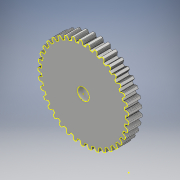
# Autodesk Inventor part: Engranaje_V_G_2
Saved by Autodesk Inventor 2017 (Build 210142000, 142)
## iProperties
Created: 2016-10-02
Part Number: Engranaje_V_G_2
Material: Generic
Document SubType Name: Modeling
Designer: CASA
Density: 1 g/cm^3
Appearance: Default
Author: CASA
Autodesk Inventor part; units mm, degrees
note: some values were not read from the file. Chosen so that the rebuilt part matches the saved one: sketch regions of "Extrusion1".
(part 1 of 2)
ref_plane "YZ Plane" through (0, 0, 0) normal (1, 0, 0) x (0, 1, 0)
ref_plane "XZ Plane" through (0, 0, 0) normal (0, 1, 0) x (-1, 0, 0)
ref_plane "XY Plane" through (0, 0, 0) normal (0, 0, 1) x (1, 0, 0)
sketch "Sketch1" plane through (0, 0, 0) normal (0, 1, 0) x (-1, 0, 0)
  line L0 (1.1447, 1.0054) -> (1.14, 0.9694)
  line L1 (1.14, 0.9694) -> (1.1261, 0.9358)
  line L2 (1.1261, 0.9358) -> (1.104, 0.907)
  line L3 (1.104, 0.907) -> (1.0751, 0.8848)
  line L4 (1.0751, 0.8848) -> (1.0415, 0.8709)
  line L5 (1.0415, 0.8709) -> (1.0055, 0.8662)
  line L6 (1.0055, 0.8662) -> (0.9694, 0.8709)
  line L7 (0.9694, 0.8709) -> (0.9358, 0.8848)
  line L8 (0.9358, 0.8848) -> (0.907, 0.907)
  line L9 (0.907, 0.907) -> (0.8848, 0.9358)
  line L10 (0.8848, 0.9358) -> (0.8709, 0.9694)
  line L11 (0.8709, 0.9694) -> (0.8662, 1.0055)
  line L12 (0.8662, 1.0055) -> (0.8709, 1.0415)
  line L13 (0.8709, 1.0415) -> (0.8848, 1.0751)
  line L14 (0.8848, 1.0751) -> (0.907, 1.104)
  line L15 (0.907, 1.104) -> (0.9358, 1.1261)
  line L16 (0.9358, 1.1261) -> (0.9694, 1.14)
  line L17 (0.9694, 1.14) -> (1.0055, 1.1447)
  line L18 (1.0055, 1.1447) -> (1.0415, 1.14)
  line L19 (1.0415, 1.14) -> (1.0751, 1.1261)
  line L20 (1.0751, 1.1261) -> (1.104, 1.104)
  line L21 (1.104, 1.104) -> (1.1261, 1.0751)
  line L22 (1.1261, 1.0751) -> (1.14, 1.0415)
  line L23 (1.14, 1.0415) -> (1.1447, 1.0054)
  line L24 (1.935, 1.0367) -> (1.9383, 1.036)
  line L25 (1.9383, 1.036) -> (1.9449, 1.0346)
  line L26 (1.9449, 1.0346) -> (1.9582, 1.0311)
  line L27 (1.9582, 1.0311) -> (1.9714, 1.0269)
  line L28 (1.9714, 1.0269) -> (1.9846, 1.0221)
  line L29 (1.9846, 1.0221) -> (1.9978, 1.0168)
  line L30 (1.9978, 1.0168) -> (2.0109, 1.0108)
  line L31 (2.0109, 1.0108) -> (2.0098, 0.9593)
  line L32 (2.0098, 0.9593) -> (1.9964, 0.9539)
  line L33 (1.9964, 0.9539) -> (1.983, 0.9491)
  line L34 (1.983, 0.9491) -> (1.9696, 0.9449)
  line L35 (1.9696, 0.9449) -> (1.9562, 0.9412)
  line L36 (1.9562, 0.9412) -> (1.9429, 0.9383)
  line L37 (1.9429, 0.9383) -> (1.9362, 0.9371)
  line L38 (1.9362, 0.9371) -> (1.9329, 0.9366)
  line L39 (1.9329, 0.9366) -> (1.9296, 0.9361)
  line L40 (1.9296, 0.9361) -> (1.9237, 0.8803)
  line L41 (1.9237, 0.8803) -> (1.9268, 0.8792)
  line L42 (1.9268, 0.8792) -> (1.93, 0.878)
  line L43 (1.93, 0.878) -> (1.9363, 0.8754)
  line L44 (1.9363, 0.8754) -> (1.9487, 0.8698)
  line L45 (1.9487, 0.8698) -> (1.961, 0.8634)
  line L46 (1.961, 0.8634) -> (1.9732, 0.8565)
  line L47 (1.9732, 0.8565) -> (1.9853, 0.849)
  line L48 (1.9853, 0.849) -> (1.9973, 0.8409)
  line L49 (1.9973, 0.8409) -> (1.9876, 0.7902)
  line L50 (1.9876, 0.7902) -> (1.9735, 0.7872)
  line L51 (1.9735, 0.7872) -> (1.9595, 0.7847)
  line L52 (1.9595, 0.7847) -> (1.9455, 0.7828)
  line L53 (1.9455, 0.7828) -> (1.9317, 0.7815)
  line L54 (1.9317, 0.7815) -> (1.9181, 0.7808)
  line L55 (1.9181, 0.7808) -> (1.9113, 0.7808)
  line L56 (1.9113, 0.7808) -> (1.9079, 0.7808)
  line L57 (1.9079, 0.7808) -> (1.9046, 0.7809)
  line L58 (1.9046, 0.7809) -> (1.8893, 0.727)
  line L59 (1.8893, 0.727) -> (1.8923, 0.7253)
  line L60 (1.8923, 0.7253) -> (1.8952, 0.7236)
  line L61 (1.8952, 0.7236) -> (1.9009, 0.72)
  line L62 (1.9009, 0.72) -> (1.9122, 0.7123)
  line L63 (1.9122, 0.7123) -> (1.9233, 0.704)
  line L64 (1.9233, 0.704) -> (1.9342, 0.6951)
  line L65 (1.9342, 0.6951) -> (1.9448, 0.6856)
  line L66 (1.9448, 0.6856) -> (1.9553, 0.6757)
  line L67 (1.9553, 0.6757) -> (1.9371, 0.6273)
  line L68 (1.9371, 0.6273) -> (1.9226, 0.6267)
  line L69 (1.9226, 0.6267) -> (1.9084, 0.6267)
  line L70 (1.9084, 0.6267) -> (1.8944, 0.6271)
  line L71 (1.8944, 0.6271) -> (1.8805, 0.6282)
  line L72 (1.8805, 0.6282) -> (1.8669, 0.6298)
  line L73 (1.8669, 0.6298) -> (1.8603, 0.6309)
  line L74 (1.8603, 0.6309) -> (1.857, 0.6316)
  line L75 (1.857, 0.6316) -> (1.8537, 0.6322)
  line L76 (1.8537, 0.6322) -> (1.8295, 0.5816)
  line L77 (1.8295, 0.5816) -> (1.8321, 0.5795)
  line L78 (1.8321, 0.5795) -> (1.8347, 0.5773)
  line L79 (1.8347, 0.5773) -> (1.8397, 0.5728)
  line L80 (1.8397, 0.5728) -> (1.8496, 0.5633)
  line L81 (1.8496, 0.5633) -> (1.8591, 0.5532)
  line L82 (1.8591, 0.5532) -> (1.8683, 0.5426)
  line L83 (1.8683, 0.5426) -> (1.8772, 0.5315)
  line L84 (1.8772, 0.5315) -> (1.8858, 0.5199)
  line L85 (1.8858, 0.5199) -> (1.8597, 0.4753)
  line L86 (1.8597, 0.4753) -> (1.8454, 0.4772)
  line L87 (1.8454, 0.4772) -> (1.8314, 0.4795)
  line L88 (1.8314, 0.4795) -> (1.8176, 0.4823)
  line L89 (1.8176, 0.4823) -> (1.8042, 0.4857)
  line L90 (1.8042, 0.4857) -> (1.7911, 0.4896)
  line L91 (1.7911, 0.4896) -> (1.7847, 0.4919)
  line L92 (1.7847, 0.4919) -> (1.7815, 0.493)
  line L93 (1.7815, 0.493) -> (1.7784, 0.4942)
  line L94 (1.7784, 0.4942) -> (1.746, 0.4484)
  line L95 (1.746, 0.4484) -> (1.7482, 0.4459)
  line L96 (1.7482, 0.4459) -> (1.7504, 0.4433)
  line L97 (1.7504, 0.4433) -> (1.7546, 0.438)
  line L98 (1.7546, 0.438) -> (1.7627, 0.427)
  line L99 (1.7627, 0.427) -> (1.7704, 0.4154)
  line L100 (1.7704, 0.4154) -> (1.7776, 0.4034)
  line L101 (1.7776, 0.4034) -> (1.7845, 0.391)
  line L102 (1.7845, 0.391) -> (1.7911, 0.3781)
  line L103 (1.7911, 0.3781) -> (1.7578, 0.3386)
  line L104 (1.7578, 0.3386) -> (1.744, 0.3428)
  line L105 (1.744, 0.3428) -> (1.7306, 0.3475)
  line L106 (1.7306, 0.3475) -> (1.7175, 0.3526)
  line L107 (1.7175, 0.3526) -> (1.7048, 0.3582)
  line L108 (1.7048, 0.3582) -> (1.6926, 0.3643)
  line L109 (1.6926, 0.3643) -> (1.6866, 0.3676)
  line L110 (1.6866, 0.3676) -> (1.6837, 0.3692)
  line L111 (1.6837, 0.3692) -> (1.6808, 0.371)
  line L112 (1.6808, 0.371) -> (1.6412, 0.3313)
  line L113 (1.6412, 0.3313) -> (1.6429, 0.3284)
  line L114 (1.6429, 0.3284) -> (1.6446, 0.3255)
  line L115 (1.6446, 0.3255) -> (1.6479, 0.3196)
  line L116 (1.6479, 0.3196) -> (1.654, 0.3073)
  line L117 (1.654, 0.3073) -> (1.6596, 0.2947)
  line L118 (1.6596, 0.2947) -> (1.6648, 0.2816)
  line L119 (1.6648, 0.2816) -> (1.6695, 0.2681)
  line L120 (1.6695, 0.2681) -> (1.6737, 0.2543)
  line L121 (1.6737, 0.2543) -> (1.6343, 0.221)
  line L122 (1.6343, 0.221) -> (1.6214, 0.2275)
  line L123 (1.6214, 0.2275) -> (1.6089, 0.2344)
  line L124 (1.6089, 0.2344) -> (1.5969, 0.2417)
  line L125 (1.5969, 0.2417) -> (1.5853, 0.2493)
  line L126 (1.5853, 0.2493) -> (1.5743, 0.2574)
  line L127 (1.5743, 0.2574) -> (1.569, 0.2616)
  line L128 (1.569, 0.2616) -> (1.5664, 0.2638)
  line L129 (1.5664, 0.2638) -> (1.5639, 0.266)
  line L130 (1.5639, 0.266) -> (1.5181, 0.2335)
  line L131 (1.5181, 0.2335) -> (1.5193, 0.2304)
  line L132 (1.5193, 0.2304) -> (1.5205, 0.2273)
  line L133 (1.5205, 0.2273) -> (1.5227, 0.2209)
  line L134 (1.5227, 0.2209) -> (1.5267, 0.2078)
  line L135 (1.5267, 0.2078) -> (1.5301, 0.1943)
  line L136 (1.5301, 0.1943) -> (1.5329, 0.1806)
  line L137 (1.5329, 0.1806) -> (1.5353, 0.1665)
  line L138 (1.5353, 0.1665) -> (1.5372, 0.1522)
  line L139 (1.5372, 0.1522) -> (1.4927, 0.126)
  line L140 (1.4927, 0.126) -> (1.4811, 0.1346)
  line L141 (1.4811, 0.1346) -> (1.4699, 0.1435)
  line L142 (1.4699, 0.1435) -> (1.4593, 0.1527)
  line L143 (1.4593, 0.1527) -> (1.4492, 0.1622)
  line L144 (1.4492, 0.1622) -> (1.4397, 0.172)
  line L145 (1.4397, 0.172) -> (1.4352, 0.1771)
  line L146 (1.4352, 0.1771) -> (1.433, 0.1796)
  line L147 (1.433, 0.1796) -> (1.4309, 0.1822)
  line L148 (1.4309, 0.1822) -> (1.3803, 0.158)
  line L149 (1.3803, 0.158) -> (1.3809, 0.1547)
  line L150 (1.3809, 0.1547) -> (1.3816, 0.1514)
  line L151 (1.3816, 0.1514) -> (1.3827, 0.1447)
  line L152 (1.3827, 0.1447) -> (1.3844, 0.1312)
  line L153 (1.3844, 0.1312) -> (1.3854, 0.1173)
  line L154 (1.3854, 0.1173) -> (1.3859, 0.1033)
  line L155 (1.3859, 0.1033) -> (1.3859, 0.089)
  line L156 (1.3859, 0.089) -> (1.3853, 0.0746)
  line L157 (1.3853, 0.0746) -> (1.337, 0.0563)
  line L158 (1.337, 0.0563) -> (1.327, 0.0668)
  line L159 (1.327, 0.0668) -> (1.3176, 0.0774)
  line L160 (1.3176, 0.0774) -> (1.3086, 0.0883)
  line L161 (1.3086, 0.0883) -> (1.3003, 0.0993)
  line L162 (1.3003, 0.0993) -> (1.2926, 0.1106)
  line L163 (1.2926, 0.1106) -> (1.289, 0.1164)
  line L164 (1.289, 0.1164) -> (1.2873, 0.1193)
  line L165 (1.2873, 0.1193) -> (1.2856, 0.1222)
  line L166 (1.2856, 0.1222) -> (1.2316, 0.1068)
  line L167 (1.2316, 0.1068) -> (1.2318, 0.1035)
  line L168 (1.2318, 0.1035) -> (1.2318, 0.1001)
  line L169 (1.2318, 0.1001) -> (1.2318, 0.0934)
  line L170 (1.2318, 0.0934) -> (1.2312, 0.0797)
  line L171 (1.2312, 0.0797) -> (1.2299, 0.0659)
  line L172 (1.2299, 0.0659) -> (1.228, 0.052)
  line L173 (1.228, 0.052) -> (1.2255, 0.0379)
  line L174 (1.2255, 0.0379) -> (1.2225, 0.0238)
  line L175 (1.2225, 0.0238) -> (1.1718, 0.014)
  line L176 (1.1718, 0.014) -> (1.1638, 0.0259)
  line L177 (1.1638, 0.0259) -> (1.1562, 0.038)
  line L178 (1.1562, 0.038) -> (1.1492, 0.0502)
  line L179 (1.1492, 0.0502) -> (1.1429, 0.0625)
  line L180 (1.1429, 0.0625) -> (1.1372, 0.075)
  line L181 (1.1372, 0.075) -> (1.1346, 0.0812)
  line L182 (1.1346, 0.0812) -> (1.1334, 0.0844)
  line L183 (1.1334, 0.0844) -> (1.1323, 0.0875)
  line L184 (1.1323, 0.0875) -> (1.0765, 0.0815)
  line L185 (1.0765, 0.0815) -> (1.076, 0.0782)
  line L186 (1.076, 0.0782) -> (1.0755, 0.0749)
  line L187 (1.0755, 0.0749) -> (1.0744, 0.0682)
  line L188 (1.0744, 0.0682) -> (1.0714, 0.0548)
  line L189 (1.0714, 0.0548) -> (1.0678, 0.0415)
  line L190 (1.0678, 0.0415) -> (1.0636, 0.028)
  line L191 (1.0636, 0.028) -> (1.0588, 0.0146)
  line L192 (1.0588, 0.0146) -> (1.0535, 0.0012)
  line L193 (1.0535, 0.0012) -> (1.0019, 0.0001)
  line L194 (1.0019, 0.0001) -> (0.9959, 0.0132)
  line L195 (0.9959, 0.0132) -> (0.9905, 0.0264)
  line L196 (0.9905, 0.0264) -> (0.9857, 0.0396)
  line L197 (0.9857, 0.0396) -> (0.9815, 0.0528)
  line L198 (0.9815, 0.0528) -> (0.978, 0.0661)
  line L199 (0.978, 0.0661) -> (0.9765, 0.0727)
  line L200 (0.9765, 0.0727) -> (0.9759, 0.076)
  line L201 (0.9759, 0.076) -> (0.9753, 0.0793)
  line L202 (0.9753, 0.0793) -> (0.9193, 0.0828)
  line L203 (0.9193, 0.0828) -> (0.9183, 0.0796)
  line L204 (0.9183, 0.0796) -> (0.9172, 0.0764)
  line L205 (0.9172, 0.0764) -> (0.9149, 0.07)
  line L206 (0.9149, 0.07) -> (0.9098, 0.0573)
  line L207 (0.9098, 0.0573) -> (0.904, 0.0448)
  line L208 (0.904, 0.0448) -> (0.8976, 0.0323)
  line L209 (0.8976, 0.0323) -> (0.8906, 0.0198)
  line L210 (0.8906, 0.0198) -> (0.883, 0.0075)
  line L211 (0.883, 0.0075) -> (0.832, 0.0151)
  line L212 (0.832, 0.0151) -> (0.8284, 0.0291)
  line L213 (0.8284, 0.0291) -> (0.8253, 0.043)
  line L214 (0.8253, 0.043) -> (0.8228, 0.0568)
  line L215 (0.8228, 0.0568) -> (0.8209, 0.0706)
  line L216 (0.8209, 0.0706) -> (0.8197, 0.0842)
  line L217 (0.8197, 0.0842) -> (0.8193, 0.0909)
  line L218 (0.8193, 0.0909) -> (0.8192, 0.0943)
  line L219 (0.8192, 0.0943) -> (0.8192, 0.0977)
  line L220 (0.8192, 0.0977) -> (0.7646, 0.1106)
  line L221 (0.7646, 0.1106) -> (0.7631, 0.1076)
  line L222 (0.7631, 0.1076) -> (0.7615, 0.1046)
  line L223 (0.7615, 0.1046) -> (0.7581, 0.0987)
  line L224 (0.7581, 0.0987) -> (0.751, 0.0871)
  line L225 (0.751, 0.0871) -> (0.7431, 0.0757)
  line L226 (0.7431, 0.0757) -> (0.7347, 0.0645)
  line L227 (0.7347, 0.0645) -> (0.7257, 0.0534)
  line L228 (0.7257, 0.0534) -> (0.7161, 0.0426)
  line L229 (0.7161, 0.0426) -> (0.6671, 0.0587)
  line L230 (0.6671, 0.0587) -> (0.6659, 0.0731)
  line L231 (0.6659, 0.0731) -> (0.6652, 0.0873)
  line L232 (0.6652, 0.0873) -> (0.6651, 0.1013)
  line L233 (0.6651, 0.1013) -> (0.6655, 0.1152)
  line L234 (0.6655, 0.1152) -> (0.6666, 0.1288)
  line L235 (0.6666, 0.1288) -> (0.6674, 0.1355)
  line L236 (0.6674, 0.1355) -> (0.6679, 0.1389)
  line L237 (0.6679, 0.1389) -> (0.6684, 0.1422)
  line L238 (0.6684, 0.1422) -> (0.6168, 0.1641)
  line L239 (0.6168, 0.1641) -> (0.6148, 0.1615)
  line L240 (0.6148, 0.1615) -> (0.6127, 0.1588)
  line L241 (0.6127, 0.1588) -> (0.6085, 0.1536)
  line L242 (0.6085, 0.1536) -> (0.5994, 0.1433)
  line L243 (0.5994, 0.1433) -> (0.5897, 0.1334)
  line L244 (0.5897, 0.1334) -> (0.5795, 0.1238)
  line L245 (0.5795, 0.1238) -> (0.5688, 0.1144)
  line L246 (0.5688, 0.1144) -> (0.5576, 0.1053)
  line L247 (0.5576, 0.1053) -> (0.512, 0.1294)
  line L248 (0.512, 0.1294) -> (0.5132, 0.1438)
  line L249 (0.5132, 0.1438) -> (0.5149, 0.158)
  line L250 (0.5149, 0.158) -> (0.5172, 0.1718)
  line L251 (0.5172, 0.1718) -> (0.5199, 0.1854)
  line L252 (0.5199, 0.1854) -> (0.5233, 0.1987)
  line L253 (0.5233, 0.1987) -> (0.5253, 0.2052)
  line L254 (0.5253, 0.2052) -> (0.5263, 0.2084)
  line L255 (0.5263, 0.2084) -> (0.5274, 0.2115)
  line L256 (0.5274, 0.2115) -> (0.4802, 0.2419)
  line L257 (0.4802, 0.2419) -> (0.4778, 0.2396)
  line L258 (0.4778, 0.2396) -> (0.4753, 0.2373)
  line L259 (0.4753, 0.2373) -> (0.4702, 0.2329)
  line L260 (0.4702, 0.2329) -> (0.4595, 0.2243)
  line L261 (0.4595, 0.2243) -> (0.4483, 0.2162)
  line L262 (0.4483, 0.2162) -> (0.4366, 0.2084)
  line L263 (0.4366, 0.2084) -> (0.4244, 0.201)
  line L264 (0.4244, 0.201) -> (0.4119, 0.1939)
  line L265 (0.4119, 0.1939) -> (0.371, 0.2254)
  line L266 (0.371, 0.2254) -> (0.3746, 0.2394)
  line L267 (0.3746, 0.2394) -> (0.3787, 0.2531)
  line L268 (0.3787, 0.2531) -> (0.3833, 0.2664)
  line L269 (0.3833, 0.2664) -> (0.3883, 0.2793)
  line L270 (0.3883, 0.2793) -> (0.3939, 0.2918)
  line L271 (0.3939, 0.2918) -> (0.3969, 0.2978)
  line L272 (0.3969, 0.2978) -> (0.3985, 0.3008)
  line L273 (0.3985, 0.3008) -> (0.4001, 0.3037)
  line L274 (0.4001, 0.3037) -> (0.3587, 0.3417)
  line L275 (0.3587, 0.3417) -> (0.3559, 0.3398)
  line L276 (0.3559, 0.3398) -> (0.3531, 0.338)
  line L277 (0.3531, 0.338) -> (0.3473, 0.3345)
  line L278 (0.3473, 0.3345) -> (0.3354, 0.3278)
  line L279 (0.3354, 0.3278) -> (0.3229, 0.3217)
  line L280 (0.3229, 0.3217) -> (0.3101, 0.316)
  line L281 (0.3101, 0.316) -> (0.2969, 0.3108)
  line L282 (0.2969, 0.3108) -> (0.2832, 0.3059)
  line L283 (0.2832, 0.3059) -> (0.2483, 0.3439)
  line L284 (0.2483, 0.3439) -> (0.2543, 0.357)
  line L285 (0.2543, 0.357) -> (0.2606, 0.3698)
  line L286 (0.2606, 0.3698) -> (0.2673, 0.3821)
  line L287 (0.2673, 0.3821) -> (0.2745, 0.394)
  line L288 (0.2745, 0.394) -> (0.2821, 0.4054)
  line L289 (0.2821, 0.4054) -> (0.2861, 0.4108)
  line L290 (0.2861, 0.4108) -> (0.2881, 0.4135)
  line L291 (0.2881, 0.4135) -> (0.2902, 0.4161)
  line L292 (0.2902, 0.4161) -> (0.2559, 0.4605)
  line L293 (0.2559, 0.4605) -> (0.2528, 0.4592)
  line L294 (0.2528, 0.4592) -> (0.2497, 0.4578)
  line L295 (0.2497, 0.4578) -> (0.2434, 0.4553)
  line L296 (0.2434, 0.4553) -> (0.2305, 0.4508)
  line L297 (0.2305, 0.4508) -> (0.2172, 0.4469)
  line L298 (0.2172, 0.4469) -> (0.2036, 0.4434)
  line L299 (0.2036, 0.4434) -> (0.1896, 0.4405)
  line L300 (0.1896, 0.4405) -> (0.1754, 0.438)
  line L301 (0.1754, 0.438) -> (0.1474, 0.4814)
  line L302 (0.1474, 0.4814) -> (0.1555, 0.4933)
  line L303 (0.1555, 0.4933) -> (0.1639, 0.5048)
  line L304 (0.1639, 0.5048) -> (0.1726, 0.5158)
  line L305 (0.1726, 0.5158) -> (0.1817, 0.5263)
  line L306 (0.1817, 0.5263) -> (0.1911, 0.5363)
  line L307 (0.1911, 0.5363) -> (0.1959, 0.541)
  line L308 (0.1959, 0.541) -> (0.1984, 0.5433)
  line L309 (0.1984, 0.5433) -> (0.2009, 0.5455)
  line L310 (0.2009, 0.5455) -> (0.1745, 0.595)
  line L311 (0.1745, 0.595) -> (0.1713, 0.5942)
  line L312 (0.1713, 0.5942) -> (0.168, 0.5934)
  line L313 (0.168, 0.5934) -> (0.1614, 0.592)
  line L314 (0.1614, 0.592) -> (0.1479, 0.5898)
  line L315 (0.1479, 0.5898) -> (0.1341, 0.5881)
  line L316 (0.1341, 0.5881) -> (0.1201, 0.587)
  line L317 (0.1201, 0.587) -> (0.1059, 0.5865)
  line L318 (0.1059, 0.5865) -> (0.0915, 0.5865)
  line L319 (0.0915, 0.5865) -> (0.0712, 0.6339)
  line L320 (0.0712, 0.6339) -> (0.0812, 0.6443)
  line L321 (0.0812, 0.6443) -> (0.0914, 0.6543)
  line L322 (0.0914, 0.6543) -> (0.1018, 0.6636)
  line L323 (0.1018, 0.6636) -> (0.1125, 0.6725)
  line L324 (0.1125, 0.6725) -> (0.1235, 0.6806)
  line L325 (0.1235, 0.6806) -> (0.1291, 0.6845)
  line L326 (0.1291, 0.6845) -> (0.1319, 0.6863)
  line L327 (0.1319, 0.6863) -> (0.1347, 0.6881)
  line L328 (0.1347, 0.6881) -> (0.1171, 0.7414)
  line L329 (0.1171, 0.7414) -> (0.1138, 0.7411)
  line L330 (0.1138, 0.7411) -> (0.1104, 0.7409)
  line L331 (0.1104, 0.7409) -> (0.1037, 0.7406)
  line L332 (0.1037, 0.7406) -> (0.09, 0.7407)
  line L333 (0.09, 0.7407) -> (0.0761, 0.7414)
  line L334 (0.0761, 0.7414) -> (0.0621, 0.7427)
  line L335 (0.0621, 0.7427) -> (0.048, 0.7446)
  line L336 (0.048, 0.7446) -> (0.0338, 0.747)
  line L337 (0.0338, 0.747) -> (0.0218, 0.7972)
  line L338 (0.0218, 0.7972) -> (0.0334, 0.8057)
  line L339 (0.0334, 0.8057) -> (0.0452, 0.8138)
  line L340 (0.0452, 0.8138) -> (0.0571, 0.8213)
  line L341 (0.0571, 0.8213) -> (0.0691, 0.8282)
  line L342 (0.0691, 0.8282) -> (0.0813, 0.8344)
  line L343 (0.0813, 0.8344) -> (0.0874, 0.8372)
  line L344 (0.0874, 0.8372) -> (0.0905, 0.8385)
  line L345 (0.0905, 0.8385) -> (0.0936, 0.8398)
  line L346 (0.0936, 0.8398) -> (0.0853, 0.8953)
  line L347 (0.0853, 0.8953) -> (0.0819, 0.8956)
  line L348 (0.0819, 0.8956) -> (0.0786, 0.896)
  line L349 (0.0786, 0.896) -> (0.0719, 0.8969)
  line L350 (0.0719, 0.8969) -> (0.0584, 0.8992)
  line L351 (0.0584, 0.8992) -> (0.0449, 0.9022)
  line L352 (0.0449, 0.9022) -> (0.0313, 0.9059)
  line L353 (0.0313, 0.9059) -> (0.0177, 0.9101)
  line L354 (0.0177, 0.9101) -> (0.0041, 0.9149)
  line L355 (0.0041, 0.9149) -> (0.0008, 0.9664)
  line L356 (0.0008, 0.9664) -> (0.0137, 0.9729)
  line L357 (0.0137, 0.9729) -> (0.0266, 0.9788)
  line L358 (0.0266, 0.9788) -> (0.0396, 0.9842)
  line L359 (0.0396, 0.9842) -> (0.0526, 0.9889)
  line L360 (0.0526, 0.9889) -> (0.0657, 0.993)
  line L361 (0.0657, 0.993) -> (0.0722, 0.9948)
  line L362 (0.0722, 0.9948) -> (0.0755, 0.9955)
  line L363 (0.0755, 0.9955) -> (0.0788, 0.9963)
  line L364 (0.0788, 0.9963) -> (0.0799, 1.0524)
  line L365 (0.0799, 1.0524) -> (0.0767, 1.0533)
  line L366 (0.0767, 1.0533) -> (0.0734, 1.0542)
  line L367 (0.0734, 1.0542) -> (0.067, 1.0562)
  line L368 (0.067, 1.0562) -> (0.0541, 1.0608)
  line L369 (0.0541, 1.0608) -> (0.0413, 1.0661)
  line L370 (0.0413, 1.0661) -> (0.0285, 1.072)
  line L371 (0.0285, 1.072) -> (0.0158, 1.0784)
  line L372 (0.0158, 1.0784) -> (0.0032, 1.0854)
  line L373 (0.0032, 1.0854) -> (0.0086, 1.1368)
  line L374 (0.0086, 1.1368) -> (0.0224, 1.141)
  line L375 (0.0224, 1.141) -> (0.0362, 1.1446)
  line L376 (0.0362, 1.1446) -> (0.0499, 1.1477)
  line L377 (0.0499, 1.1477) -> (0.0635, 1.1502)
  line L378 (0.0635, 1.1502) -> (0.0771, 1.152)
  line L379 (0.0771, 1.152) -> (0.0838, 1.1526)
  line L380 (0.0838, 1.1526) -> (0.0872, 1.1529)
  line L381 (0.0872, 1.1529) -> (0.0905, 1.153)
  line L382 (0.0905, 1.153) -> (0.1011, 1.2081)
  line L383 (0.1011, 1.2081) -> (0.0981, 1.2095)
  line L384 (0.0981, 1.2095) -> (0.0951, 1.211)
  line L385 (0.0951, 1.211) -> (0.089, 1.2141)
  line L386 (0.089, 1.2141) -> (0.0771, 1.2208)
  line L387 (0.0771, 1.2208) -> (0.0654, 1.2281)
  line L388 (0.0654, 1.2281) -> (0.0538, 1.2361)
  line L389 (0.0538, 1.2361) -> (0.0424, 1.2446)
  line L390 (0.0424, 1.2446) -> (0.0311, 1.2537)
  line L391 (0.0311, 1.2537) -> (0.0451, 1.3033)
  line L392 (0.0451, 1.3033) -> (0.0595, 1.3052)
  line L393 (0.0595, 1.3052) -> (0.0736, 1.3065)
  line L394 (0.0736, 1.3065) -> (0.0877, 1.3072)
  line L395 (0.0877, 1.3072) -> (0.1015, 1.3073)
  line L396 (0.1015, 1.3073) -> (0.1152, 1.3068)
  line L397 (0.1152, 1.3068) -> (0.122, 1.3063)
  line L398 (0.122, 1.3063) -> (0.1253, 1.3059)
  line L399 (0.1253, 1.3059) -> (0.1286, 1.3055)
  line L400 (0.1286, 1.3055) -> (0.1484, 1.358)
  line L401 (0.1484, 1.358) -> (0.1456, 1.3599)
  line L402 (0.1456, 1.3599) -> (0.1429, 1.3619)
  line L403 (0.1429, 1.3619) -> (0.1375, 1.3659)
  line L404 (0.1375, 1.3659) -> (0.1269, 1.3746)
  line L405 (0.1269, 1.3746) -> (0.1165, 1.3838)
  line L406 (0.1165, 1.3838) -> (0.1065, 1.3936)
  line L407 (0.1065, 1.3936) -> (0.0966, 1.4039)
  line L408 (0.0966, 1.4039) -> (0.0871, 1.4148)
  line L409 (0.0871, 1.4148) -> (0.1093, 1.4613)
  line L410 (0.1093, 1.4613) -> (0.1237, 1.4607)
  line L411 (0.1237, 1.4607) -> (0.1379, 1.4596)
  line L412 (0.1379, 1.4596) -> (0.1519, 1.458)
  line L413 (0.1519, 1.458) -> (0.1656, 1.4557)
  line L414 (0.1656, 1.4557) -> (0.1789, 1.4529)
  line L415 (0.1789, 1.4529) -> (0.1855, 1.4513)
  line L416 (0.1855, 1.4513) -> (0.1887, 1.4504)
  line L417 (0.1887, 1.4504) -> (0.192, 1.4494)
  line L418 (0.192, 1.4494) -> (0.2203, 1.4978)
  line L419 (0.2203, 1.4978) -> (0.2179, 1.5002)
  line L420 (0.2179, 1.5002) -> (0.2155, 1.5025)
  line L421 (0.2155, 1.5025) -> (0.2109, 1.5075)
  line L422 (0.2109, 1.5075) -> (0.2019, 1.5177)
  line L423 (0.2019, 1.5177) -> (0.1933, 1.5286)
  line L424 (0.1933, 1.5286) -> (0.185, 1.54)
  line L425 (0.185, 1.54) -> (0.1771, 1.5518)
  line L426 (0.1771, 1.5518) -> (0.1695, 1.5641)
  line L427 (0.1695, 1.5641) -> (0.1992, 1.6062)
  line L428 (0.1992, 1.6062) -> (0.2133, 1.6032)
  line L429 (0.2133, 1.6032) -> (0.2271, 1.5997)
  line L430 (0.2271, 1.5997) -> (0.2406, 1.5957)
  line L431 (0.2406, 1.5957) -> (0.2537, 1.5912)
  line L432 (0.2537, 1.5912) -> (0.2665, 1.5862)
  line L433 (0.2665, 1.5862) -> (0.2726, 1.5834)
  line L434 (0.2726, 1.5834) -> (0.2757, 1.582)
  line L435 (0.2757, 1.582) -> (0.2787, 1.5805)
  line L436 (0.2787, 1.5805) -> (0.3148, 1.6234)
  line L437 (0.3148, 1.6234) -> (0.3128, 1.6261)
  line L438 (0.3128, 1.6261) -> (0.3109, 1.6289)
  line L439 (0.3109, 1.6289) -> (0.3071, 1.6345)
  line L440 (0.3071, 1.6345) -> (0.3, 1.6462)
  line L441 (0.3, 1.6462) -> (0.2933, 1.6583)
  line L442 (0.2933, 1.6583) -> (0.2871, 1.6709)
  line L443 (0.2871, 1.6709) -> (0.2813, 1.6839)
  line L444 (0.2813, 1.6839) -> (0.2759, 1.6973)
  line L445 (0.2759, 1.6973) -> (0.3123, 1.7339)
  line L446 (0.3123, 1.7339) -> (0.3257, 1.7285)
  line L447 (0.3257, 1.7285) -> (0.3388, 1.7227)
  line L448 (0.3388, 1.7227) -> (0.3514, 1.7165)
  line L449 (0.3514, 1.7165) -> (0.3635, 1.7098)
  line L450 (0.3635, 1.7098) -> (0.3752, 1.7027)
  line L451 (0.3752, 1.7027) -> (0.3809, 1.699)
  line L452 (0.3809, 1.699) -> (0.3836, 1.697)
  line L453 (0.3836, 1.697) -> (0.3863, 1.6951)
  line L454 (0.3863, 1.6951) -> (0.4292, 1.7313)
  line L455 (0.4292, 1.7313) -> (0.4277, 1.7343)
  line L456 (0.4277, 1.7343) -> (0.4263, 1.7373)
  line L457 (0.4263, 1.7373) -> (0.4235, 1.7435)
  line L458 (0.4235, 1.7435) -> (0.4184, 1.7562)
  line L459 (0.4184, 1.7562) -> (0.4139, 1.7693)
  line L460 (0.4139, 1.7693) -> (0.4099, 1.7828)
  line L461 (0.4099, 1.7828) -> (0.4064, 1.7966)
  line L462 (0.4064, 1.7966) -> (0.4033, 1.8107)
  line L463 (0.4033, 1.8107) -> (0.4454, 1.8405)
  line L464 (0.4454, 1.8405) -> (0.4577, 1.8329)
  line L465 (0.4577, 1.8329) -> (0.4696, 1.825)
  line L466 (0.4696, 1.825) -> (0.4809, 1.8168)
  line L467 (0.4809, 1.8168) -> (0.4918, 1.8082)
  line L468 (0.4918, 1.8082) -> (0.5021, 1.7992)
  line L469 (0.5021, 1.7992) -> (0.507, 1.7945)
  line L470 (0.507, 1.7945) -> (0.5094, 1.7922)
  line L471 (0.5094, 1.7922) -> (0.5118, 1.7898)
  line L472 (0.5118, 1.7898) -> (0.5601, 1.8182)
  line L473 (0.5601, 1.8182) -> (0.5592, 1.8214)
  line L474 (0.5592, 1.8214) -> (0.5583, 1.8247)
  line L475 (0.5583, 1.8247) -> (0.5566, 1.8312)
  line L476 (0.5566, 1.8312) -> (0.5537, 1.8446)
  line L477 (0.5537, 1.8446) -> (0.5515, 1.8583)
  line L478 (0.5515, 1.8583) -> (0.5498, 1.8722)
  line L479 (0.5498, 1.8722) -> (0.5487, 1.8864)
  line L480 (0.5487, 1.8864) -> (0.548, 1.9009)
  line L481 (0.548, 1.9009) -> (0.5946, 1.9232)
  line L482 (0.5946, 1.9232) -> (0.6054, 1.9136)
  line L483 (0.6054, 1.9136) -> (0.6158, 1.9038)
  line L484 (0.6158, 1.9038) -> (0.6256, 1.8938)
  line L485 (0.6256, 1.8938) -> (0.6349, 1.8834)
  line L486 (0.6349, 1.8834) -> (0.6435, 1.8728)
  line L487 (0.6435, 1.8728) -> (0.6476, 1.8674)
  line L488 (0.6476, 1.8674) -> (0.6495, 1.8647)
  line L489 (0.6495, 1.8647) -> (0.6514, 1.8619)
  line L490 (0.6514, 1.8619) -> (0.7039, 1.8818)
  line L491 (0.7039, 1.8818) -> (0.7035, 1.8851)
  line L492 (0.7035, 1.8851) -> (0.7031, 1.8885)
  line L493 (0.7031, 1.8885) -> (0.7026, 1.8952)
  line L494 (0.7026, 1.8952) -> (0.7021, 1.9089)
  line L495 (0.7021, 1.9089) -> (0.7022, 1.9227)
  line L496 (0.7022, 1.9227) -> (0.7029, 1.9368)
  line L497 (0.7029, 1.9368) -> (0.7041, 1.951)
  line L498 (0.7041, 1.951) -> (0.706, 1.9653)
  line L499 (0.706, 1.9653) -> (0.7556, 1.9794)
  line L500 (0.7556, 1.9794) -> (0.7647, 1.9682)
  line L501 (0.7647, 1.9682) -> (0.7732, 1.9567)
  line L502 (0.7732, 1.9567) -> (0.7812, 1.9452)
  line L503 (0.7812, 1.9452) -> (0.7886, 1.9334)
  line L504 (0.7886, 1.9334) -> (0.7953, 1.9215)
  line L505 (0.7953, 1.9215) -> (0.7984, 1.9155)
  line L506 (0.7984, 1.9155) -> (0.7998, 1.9125)
  line L507 (0.7998, 1.9125) -> (0.8013, 1.9094)
  line L508 (0.8013, 1.9094) -> (0.8563, 1.9201)
  line L509 (0.8563, 1.9201) -> (0.8565, 1.9235)
  line L510 (0.8565, 1.9235) -> (0.8567, 1.9268)
  line L511 (0.8567, 1.9268) -> (0.8573, 1.9336)
  line L512 (0.8573, 1.9336) -> (0.8591, 1.9471)
  line L513 (0.8591, 1.9471) -> (0.8616, 1.9608)
  line L514 (0.8616, 1.9608) -> (0.8646, 1.9745)
  line L515 (0.8646, 1.9745) -> (0.8683, 1.9883)
  line L516 (0.8683, 1.9883) -> (0.8725, 2.0021)
  line L517 (0.8725, 2.0021) -> (0.9238, 2.0076)
  line L518 (0.9238, 2.0076) -> (0.9308, 1.995)
  line L519 (0.9308, 1.995) -> (0.9373, 1.9823)
  line L520 (0.9373, 1.9823) -> (0.9432, 1.9696)
  line L521 (0.9432, 1.9696) -> (0.9485, 1.9568)
  line L522 (0.9485, 1.9568) -> (0.9531, 1.9439)
  line L523 (0.9531, 1.9439) -> (0.9552, 1.9374)
  line L524 (0.9552, 1.9374) -> (0.9561, 1.9342)
  line L525 (0.9561, 1.9342) -> (0.957, 1.931)
  line L526 (0.957, 1.931) -> (1.0131, 1.9322)
  line L527 (1.0131, 1.9322) -> (1.0138, 1.9355)
  line L528 (1.0138, 1.9355) -> (1.0146, 1.9387)
  line L529 (1.0146, 1.9387) -> (1.0163, 1.9453)
  line L530 (1.0163, 1.9453) -> (1.0203, 1.9583)
  line L531 (1.0203, 1.9583) -> (1.0251, 1.9714)
  line L532 (1.0251, 1.9714) -> (1.0304, 1.9844)
  line L533 (1.0304, 1.9844) -> (1.0363, 1.9973)
  line L534 (1.0363, 1.9973) -> (1.0428, 2.0102)
  line L535 (1.0428, 2.0102) -> (1.0943, 2.007)
  line L536 (1.0943, 2.007) -> (1.0991, 1.9934)
  line L537 (1.0991, 1.9934) -> (1.1034, 1.9798)
  line L538 (1.1034, 1.9798) -> (1.107, 1.9662)
  line L539 (1.107, 1.9662) -> (1.1101, 1.9527)
  line L540 (1.1101, 1.9527) -> (1.1125, 1.9392)
  line L541 (1.1125, 1.9392) -> (1.1134, 1.9325)
  line L542 (1.1134, 1.9325) -> (1.1138, 1.9292)
  line L543 (1.1138, 1.9292) -> (1.1141, 1.9259)
  line L544 (1.1141, 1.9259) -> (1.1696, 1.9176)
  line L545 (1.1696, 1.9176) -> (1.1708, 1.9207)
  line L546 (1.1708, 1.9207) -> (1.1722, 1.9238)
  line L547 (1.1722, 1.9238) -> (1.175, 1.9299)
  line L548 (1.175, 1.9299) -> (1.1812, 1.9421)
  line L549 (1.1812, 1.9421) -> (1.188, 1.9542)
  line L550 (1.188, 1.9542) -> (1.1955, 1.9661)
  line L551 (1.1955, 1.9661) -> (1.2035, 1.9779)
  line L552 (1.2035, 1.9779) -> (1.2121, 1.9895)
  line L553 (1.2121, 1.9895) -> (1.2623, 1.9776)
  line L554 (1.2623, 1.9776) -> (1.2647, 1.9634)
  line L555 (1.2647, 1.9634) -> (1.2666, 1.9493)
  line L556 (1.2666, 1.9493) -> (1.268, 1.9353)
  line L557 (1.268, 1.9353) -> (1.2687, 1.9214)
  line L558 (1.2687, 1.9214) -> (1.2688, 1.9077)
  line L559 (1.2688, 1.9077) -> (1.2685, 1.901)
  line L560 (1.2685, 1.901) -> (1.2683, 1.8976)
  line L561 (1.2683, 1.8976) -> (1.2681, 1.8943)
  line L562 (1.2681, 1.8943) -> (1.3214, 1.8768)
  line L563 (1.3214, 1.8768) -> (1.3231, 1.8796)
  line L564 (1.3231, 1.8796) -> (1.325, 1.8824)
  line L565 (1.325, 1.8824) -> (1.3288, 1.888)
  line L566 (1.3288, 1.888) -> (1.337, 1.899)
  line L567 (1.337, 1.899) -> (1.3458, 1.9097)
  line L568 (1.3458, 1.9097) -> (1.3551, 1.9202)
  line L569 (1.3551, 1.9202) -> (1.365, 1.9304)
  line L570 (1.365, 1.9304) -> (1.3754, 1.9405)
  line L571 (1.3754, 1.9405) -> (1.4229, 1.9202)
  line L572 (1.4229, 1.9202) -> (1.4229, 1.9058)
  line L573 (1.4229, 1.9058) -> (1.4224, 1.8916)
  line L574 (1.4224, 1.8916) -> (1.4213, 1.8776)
  line L575 (1.4213, 1.8776) -> (1.4197, 1.8638)
  line L576 (1.4197, 1.8638) -> (1.4175, 1.8503)
  line L577 (1.4175, 1.8503) -> (1.4161, 1.8437)
  line L578 (1.4161, 1.8437) -> (1.4153, 1.8404)
  line L579 (1.4153, 1.8404) -> (1.4145, 1.8371)
  line L580 (1.4145, 1.8371) -> (1.4641, 1.8109)
  line L581 (1.4641, 1.8109) -> (1.4663, 1.8134)
  line L582 (1.4663, 1.8134) -> (1.4686, 1.8158)
  line L583 (1.4686, 1.8158) -> (1.4733, 1.8207)
  line L584 (1.4733, 1.8207) -> (1.4832, 1.8301)
  line L585 (1.4832, 1.8301) -> (1.4937, 1.8392)
  line L586 (1.4937, 1.8392) -> (1.5047, 1.848)
  line L587 (1.5047, 1.848) -> (1.5162, 1.8564)
  line L588 (1.5162, 1.8564) -> (1.5281, 1.8645)
  line L589 (1.5281, 1.8645) -> (1.5715, 1.8365)
  line L590 (1.5715, 1.8365) -> (1.5691, 1.8223)
  line L591 (1.5691, 1.8223) -> (1.5661, 1.8084)
  line L592 (1.5661, 1.8084) -> (1.5627, 1.7947)
  line L593 (1.5627, 1.7947) -> (1.5588, 1.7814)
  line L594 (1.5588, 1.7814) -> (1.5543, 1.7685)
  line L595 (1.5543, 1.7685) -> (1.5518, 1.7622)
  line L596 (1.5518, 1.7622) -> (1.5505, 1.7591)
  line L597 (1.5505, 1.7591) -> (1.5492, 1.7561)
  line L598 (1.5492, 1.7561) -> (1.5936, 1.7218)
  line L599 (1.5936, 1.7218) -> (1.5962, 1.7239)
  line L600 (1.5962, 1.7239) -> (1.5989, 1.7259)
  line L601 (1.5989, 1.7259) -> (1.6043, 1.7299)
  line L602 (1.6043, 1.7299) -> (1.6157, 1.7375)
  line L603 (1.6157, 1.7375) -> (1.6276, 1.7447)
  line L604 (1.6276, 1.7447) -> (1.6399, 1.7515)
  line L605 (1.6399, 1.7515) -> (1.6526, 1.7578)
  line L606 (1.6526, 1.7578) -> (1.6658, 1.7638)
  line L607 (1.6658, 1.7638) -> (1.7038, 1.7289)
  line L608 (1.7038, 1.7289) -> (1.699, 1.7153)
  line L609 (1.699, 1.7153) -> (1.6938, 1.7021)
  line L610 (1.6938, 1.7021) -> (1.6881, 1.6892)
  line L611 (1.6881, 1.6892) -> (1.682, 1.6768)
  line L612 (1.682, 1.6768) -> (1.6754, 1.6648)
  line L613 (1.6754, 1.6648) -> (1.6718, 1.659)
  line L614 (1.6718, 1.659) -> (1.67, 1.6562)
  line L615 (1.67, 1.6562) -> (1.6682, 1.6534)
  line L616 (1.6682, 1.6534) -> (1.7062, 1.6121)
  line L617 (1.7062, 1.6121) -> (1.7091, 1.6137)
  line L618 (1.7091, 1.6137) -> (1.7121, 1.6153)
  line L619 (1.7121, 1.6153) -> (1.7181, 1.6183)
  line L620 (1.7181, 1.6183) -> (1.7306, 1.6239)
  line L621 (1.7306, 1.6239) -> (1.7435, 1.629)
  line L622 (1.7435, 1.629) -> (1.7568, 1.6335)
  line L623 (1.7568, 1.6335) -> (1.7705, 1.6376)
  line L624 (1.7705, 1.6376) -> (1.7844, 1.6413)
  line L625 (1.7844, 1.6413) -> (1.816, 1.6005)
  line L626 (1.816, 1.6005) -> (1.809, 1.5879)
  line L627 (1.809, 1.5879) -> (1.8016, 1.5757)
  line L628 (1.8016, 1.5757) -> (1.7938, 1.564)
  line L629 (1.7938, 1.564) -> (1.7857, 1.5528)
  line L630 (1.7857, 1.5528) -> (1.7771, 1.5421)
  line L631 (1.7771, 1.5421) -> (1.7727, 1.537)
  line L632 (1.7727, 1.537) -> (1.7704, 1.5345)
  line L633 (1.7704, 1.5345) -> (1.7682, 1.5321)
  line L634 (1.7682, 1.5321) -> (1.7986, 1.485)
  line L635 (1.7986, 1.485) -> (1.8018, 1.486)
  line L636 (1.8018, 1.486) -> (1.805, 1.4871)
  line L637 (1.805, 1.4871) -> (1.8115, 1.489)
  line L638 (1.8115, 1.489) -> (1.8247, 1.4924)
  line L639 (1.8247, 1.4924) -> (1.8383, 1.4953)
  line L640 (1.8383, 1.4953) -> (1.8522, 1.4975)
  line L641 (1.8522, 1.4975) -> (1.8663, 1.4993)
  line L642 (1.8663, 1.4993) -> (1.8807, 1.5005)
  line L643 (1.8807, 1.5005) -> (1.9049, 1.455)
  line L644 (1.9049, 1.455) -> (1.8958, 1.4437)
  line L645 (1.8958, 1.4437) -> (1.8865, 1.433)
  line L646 (1.8865, 1.433) -> (1.8769, 1.4227)
  line L647 (1.8769, 1.4227) -> (1.867, 1.4131)
  line L648 (1.867, 1.4131) -> (1.8567, 1.404)
  line L649 (1.8567, 1.404) -> (1.8515, 1.3997)
  line L650 (1.8515, 1.3997) -> (1.8488, 1.3976)
  line L651 (1.8488, 1.3976) -> (1.8462, 1.3956)
  line L652 (1.8462, 1.3956) -> (1.8682, 1.344)
  line L653 (1.8682, 1.344) -> (1.8715, 1.3446)
  line L654 (1.8715, 1.3446) -> (1.8749, 1.345)
  line L655 (1.8749, 1.345) -> (1.8816, 1.3459)
  line L656 (1.8816, 1.3459) -> (1.8952, 1.347)
  line L657 (1.8952, 1.347) -> (1.9091, 1.3475)
  line L658 (1.9091, 1.3475) -> (1.9231, 1.3474)
  line L659 (1.9231, 1.3474) -> (1.9374, 1.3467)
  line L660 (1.9374, 1.3467) -> (1.9517, 1.3455)
  line L661 (1.9517, 1.3455) -> (1.9679, 1.2965)
  line L662 (1.9679, 1.2965) -> (1.9571, 1.287)
  line L663 (1.9571, 1.287) -> (1.9461, 1.278)
  line L664 (1.9461, 1.278) -> (1.9349, 1.2695)
  line L665 (1.9349, 1.2695) -> (1.9234, 1.2616)
  line L666 (1.9234, 1.2616) -> (1.9118, 1.2544)
  line L667 (1.9118, 1.2544) -> (1.9059, 1.251)
  line L668 (1.9059, 1.251) -> (1.903, 1.2495)
  line L669 (1.903, 1.2495) -> (1.9, 1.2479)
  line L670 (1.9, 1.2479) -> (1.913, 1.1933)
  line L671 (1.913, 1.1933) -> (1.9164, 1.1933)
  line L672 (1.9164, 1.1933) -> (1.9197, 1.1932)
  line L673 (1.9197, 1.1932) -> (1.9265, 1.1929)
  line L674 (1.9265, 1.1929) -> (1.9401, 1.1917)
  line L675 (1.9401, 1.1917) -> (1.9539, 1.1898)
  line L676 (1.9539, 1.1898) -> (1.9677, 1.1874)
  line L677 (1.9677, 1.1874) -> (1.9816, 1.1843)
  line L678 (1.9816, 1.1843) -> (1.9956, 1.1807)
  line L679 (1.9956, 1.1807) -> (2.0033, 1.1297)
  line L680 (2.0033, 1.1297) -> (1.991, 1.1221)
  line L681 (1.991, 1.1221) -> (1.9786, 1.1151)
  line L682 (1.9786, 1.1151) -> (1.9661, 1.1086)
  line L683 (1.9661, 1.1086) -> (1.9535, 1.1028)
  line L684 (1.9535, 1.1028) -> (1.9408, 1.0976)
  line L685 (1.9408, 1.0976) -> (1.9345, 1.0953)
  line L686 (1.9345, 1.0953) -> (1.9313, 1.0943)
  line L687 (1.9313, 1.0943) -> (1.9281, 1.0933)
  line L688 (1.9281, 1.0933) -> (1.9317, 1.0373)
  line L689 (1.9317, 1.0373) -> (1.935, 1.0367)
  line L690 (0, 0) -> (2.0109, 0)
  line L691 (2.0109, 0) -> (2.0109, 1.0108)
  line L692 (2.0109, 1.0108) -> (0, 1.0108)
  line L693 (0, 1.0108) -> (0, 0)
  line L694 (2.0109, 0) -> (-0.7541, 2.765)
  line L695 (2.0109, 0) -> (5.9212, 0) construction
  line L696 (0, 0) -> (3.1444, 3.1444)
  line L697 (0, 0) -> (4.4469, 0) construction
  circle A0 centre (1.0054, 1.0054) radius 0.13
  dimension "d2" = 135
  dimension "d3" = 45
  dimension "d4" = 0.26
  constraints: 1396 end point, 36 parallel, 32 perpendicular, 3 horizontal, 2 equal length, 2 point on line, 1 centre point
  measures "d2" angle of L695 L694
  measures "d3" angle of L697 L696
  measures "d4" diameter of A0
extrude "Extrusion1" add sketch "Sketch1" along normal blind 0.3 contours L23 L692 L31 L32 L33 L34 L35 L36 L37 L38 L39 L40 L41 L42 L43 L44 L45 L46 L47 L48 L49 L50 L51 L52 L53 L54 L55 L56 L57 L58 L59 L60 L61 L62 L63 L64 L65 L66 L67 L68 L69 L70 L71 L72 L73 L74 L75 L76 L77 L78 L79 L80 L81 L82 L83 L84 L85 L86 L87 L88 L89 L90 L91 L92 L93 L94 L95 L96 L97 L98 L99 L100 L101 L102 L103 L104 L105 L106 L107 L108 L109 L110 L111 L112 L694 L2 L1 L0 | L0 L1 L2 L694 A0 L692 L23 | L692 A0 L696 L21 L22 L23 | L23 L22 L21 L696 L611 L612 L613 L614 L615 L616 L617 L618 L619 L620 L621 L622 L623 L624 L625 L626 L627 L628 L629 L630 L631 L632 L633 L634 L635 L636 L637 L638 L639 L640 L641 L642 L643 L644 L645 L646 L647 L648 L649 L650 L651 L652 L653 L654 L655 L656 L657 L658 L659 L660 L661 L662 L663 L664 L665 L666 L667 L668 L669 L670 L671 L672 L673 L674 L675 L676 L677 L678 L679 L680 L681 L682 L683 L684 L685 L686 L687 L688 L689 L24 L25 L26 L27 L28 L29 L30 L692 | L694 L112 L113 L114 L115 L116 L117 L118 L119 L120 L121 L122 L123 L124 L125 L126 L127 L128 L129 L130 L131 L132 L133 L134 L135 L136 L137 L138 L139 L140 L141 L142 L143 L144 L145 L146 L147 L148 L149 L150 L151 L152 L153 L154 L155 L156 L157 L158 L159 L160 L161 L162 L163 L164 L165 L166 L167 L168 L169 L170 L171 L172 L173 L174 L175 L176 L177 L178 L179 L180 L181 L182 L183 L184 L185 L186 L187 L188 L189 L190 L191 L192 L193 L194 L195 L196 L197 L198 L199 L200 L201 L202 L203 L204 L205 L206 L207 L208 L209 L210 L211 L212 L213 L214 L215 L216 L217 L218 L219 L220 L221 L222 L223 L224 L225 L226 L227 L228 L229 L230 L231 L232 L233 L234 L235 L236 L237 L238 L239 L240 L241 L242 L243 L244 L245 L246 L247 L248 L249 L250 L251 L252 L253 L254 L255 L256 L257 L258 L259 L260 L261 L262 L263 L264 L265 L266 L267 L268 L269 L270 L271 L272 L273 L274 L275 L276 L277 L278 L279 L696 L8 L7 L6 L5 L4 L3 | L3 L4 L5 L6 L7 L8 L696 A0 L694 | A0 L694 L15 L16 L17 L18 L19 L20 L696 | L20 L19 L18 L17 L16 L15 L694 L445 L446 L447 L448 L449 L450 L451 L452 L453 L454 L455 L456 L457 L458 L459 L460 L461 L462 L463 L464 L465 L466 L467 L468 L469 L470 L471 L472 L473 L474 L475 L476 L477 L478 L479 L480 L481 L482 L483 L484 L485 L486 L487 L488 L489 L490 L491 L492 L493 L494 L495 L496 L497 L498 L499 L500 L501 L502 L503 L504 L505 L506 L507 L508 L509 L510 L511 L512 L513 L514 L515 L516 L517 L518 L519 L520 L521 L522 L523 L524 L525 L526 L527 L528 L529 L530 L531 L532 L533 L534 L535 L536 L537 L538 L539 L540 L541 L542 L543 L544 L545 L546 L547 L548 L549 L550 L551 L552 L553 L554 L555 L556 L557 L558 L559 L560 L561 L562 L563 L564 L565 L566 L567 L568 L569 L570 L571 L572 L573 L574 L575 L576 L577 L578 L579 L580 L581 L582 L583 L584 L585 L586 L587 L588 L589 L590 L591 L592 L593 L594 L595 L596 L597 L598 L599 L600 L601 L602 L603 L604 L605 L606 L607 L608 L609 L610 L696 | A0 L692 L12 L13 L14 L694 | L696 L9 L10 L11 L12 L692 A0 | L14 L13 L12 L692 L364 L365 L366 L367 L368 L369 L370 L371 L372 L373 L374 L375 L376 L377 L378 L379 L380 L381 L382 L383 L384 L385 L386 L387 L388 L389 L390 L391 L392 L393 L394 L395 L396 L397 L398 L399 L400 L401 L402 L403 L404 L405 L406 L407 L408 L409 L410 L411 L412 L413 L414 L415 L416 L417 L418 L419 L420 L421 L422 L423 L424 L425 L426 L427 L428 L429 L430 L431 L432 L433 L434 L435 L436 L437 L438 L439 L440 L441 L442 L443 L444 L445 L694 | L696 L280 L281 L282 L283 L284 L285 L286 L287 L288 L289 L290 L291 L292 L293 L294 L295 L296 L297 L298 L299 L300 L301 L302 L303 L304 L305 L306 L307 L308 L309 L310 L311 L312 L313 L314 L315 L316 L317 L318 L319 L320 L321 L322 L323 L324 L325 L326 L327 L328 L329 L330 L331 L332 L333 L334 L335 L336 L337 L338 L339 L340 L341 L342 L343 L344 L345 L346 L347 L348 L349 L350 L351 L352 L353 L354 L355 L356 L357 L358 L359 L360 L361 L362 L363 L364 L692 L12 L11 L10 L9